25TServoHorn (Autodesk Fusion 360 design; units mm, degrees)
Autodesk Fusion 360 part; units mm, degrees
note: some values were not read from the file. Set by a fixed rule: which sketch regions a step uses.
sketch "Sketch1" plane through (0, 0, 0) normal (0, 1, 0) x (1, 0, 0)
  circle A0 centre (0, 0) radius 10
  circle A1 centre (0, 0) radius 4.5
  circle A2 centre (0, 0) radius 2.75
  circle A3 centre (0, 0) radius 1.5
  dimension "d1" = 20
  dimension "d2" = 9
  dimension "d3" = 5.5
  dimension "d4" = 3
  constraint coincident A0.centre A1.centre
  constraint concentric A1 A2
  measures "d1" diameter of A0
  measures "d2" diameter of A1
  measures "d3" diameter of A2
  measures "d4" diameter of A3
extrude "Extrude1" add sketch "Sketch1" along normal blind 2 contours A0
extrude "Extrude2" add sketch "Sketch1" along normal blind 4.5 contours A1
extrude "Extrude3" add sketch "Sketch1" along normal blind 1 contours A2
sketch "Sketch2" plane through (0, 2, 0) normal (0, 1, 0) x (-1, 0, 0)
  circle A0 centre (0, 0) radius 4.5
  circle A1 centre (0, 0) radius 10
  circle A2 centre (0, 0) radius 7
  circle A3 centre (7, 0) radius 1.5
  line L0 (0, 0) -> (10, 0) construction
  dimension "d11" = 14
  dimension "d12" = 3
  constraint concentric A0 A2
  constraint coincident A2 A3.centre
  constraint coincident A0.centre A1.centre
  constraint coincident A1 L0.end
  constraint horizontal L0
  constraint coincident A3.centre L0
  measures "d11" diameter of A2
  measures "d12" diameter of A3
extrude "Extrude4" cut sketch "Sketch2" against normal up to surface (2 mm away) contours A2 A3 | A2 A3 picked at (6.5153, -0.3111) picked at (7.4507, -0.3705)
pattern_circular "C-Pattern1" count 4 over 360 about axis through (0, 1.75, 0) along (0, 1, 0) of "Extrude4"
sketch "Sketch3" plane through (0, 4.5, 0) normal (0, 1, 0) x (-1, 0, 0)
  circle A0 centre (0, 0) radius 2.75
  circle A1 centre (0, 0) radius 4.5
  circle A2 centre (0, 0) radius 3
  line L0 (0, 0) -> (3, 0)
  line L1 (0, 0) -> (2.9763, -0.376)
  line L2 (0, 0) -> (2.9057, -0.7461)
  line L3 (2.6636, -0.6839) -> (2.9763, -0.376)
  line L4 (2.75, 0) -> (2.9763, -0.376)
  dimension "d17" = 6
  dimension "d18" = 7.2
  dimension "d19" = 14.4
  constraint concentric A0 A2
  constraint coincident A0.centre A1.centre
  constraint coincident A2 L0.end
  constraint horizontal L0
  constraint coincident A2 L1.end
  constraint coincident A2 L2.end
  constraint coincident L2 L3.start
  constraint coincident A0 L3.start
  constraint coincident L0 L4.start
  constraint coincident A0 L4.start
  measures "d17" diameter of A2
  measures "d18" angle of L0 L1
  measures "d19" angle of L0 L2
extrude "Extrude5" cut sketch "Sketch3" against normal up to surface (3.5 mm away) contours A0 L1 L4 | A0 L1 L3
pattern_circular "C-Pattern2" count 25 over 360 about axis through (0, 1.75, 0) along (0, 1, 0) of "Extrude5"
